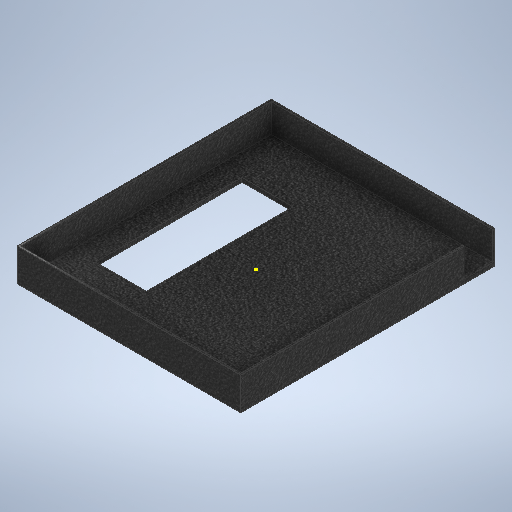
# Autodesk Inventor part: kotak_v2
Saved by Autodesk Inventor 2025.2 (Build 292293000, 293)
## iProperties
Created: 2025-02-11
Part Number: kotak_v2
Material: Generic
Document SubType Name: Modeling
Designer: ACER
Density: 1 g/cm^3
Appearance: Black Cast
Author: ACER
Autodesk Inventor part; units mm, degrees
ref_plane "YZ Plane" through (0, 0, 0) normal (1, 0, 0) x (0, 1, 0)
ref_plane "XZ Plane" through (0, 0, 0) normal (0, 1, 0) x (-1, 0, 0)
ref_plane "XY Plane" through (0, 0, 0) normal (0, 0, 1) x (1, 0, 0)
sketch "Sketch1" plane through (0, 0, 0) normal (0, 1, 0) x (-1, 0, 0)
  line L0 (-55, 62.5) -> (55, 62.5)
  line L1 (55, 62.5) -> (55, -62.5)
  line L2 (55, -62.5) -> (-55, -62.5)
  line L3 (-55, -62.5) -> (-55, 62.5)
  line L4 (-55, 62.5) -> (55, -62.5) construction
  line L5 (55, 62.5) -> (-55, -62.5) construction
  point P0 (0, 0)
  dimension "d0" = 125
  dimension "d1" = 110
  constraints: 12 end point, 2 midpoint, 2 parallel, 1 horizontal, 1 perpendicular
  measures "d0" distance of L0.end L1.end
  measures "d1" distance of L0.start L0.end
extrude "Extrusion1" add sketch "Sketch1" along normal blind 16
sketch "Sketch2" plane through (0, 16, 0) normal (0, 1, 0) x (1, 0, 0)
  line L0 (54, -61.5) -> (-54, -61.5)
  line L1 (-54, -61.5) -> (-54, 61.5)
  line L2 (-54, 61.5) -> (54, 61.5)
  line L3 (54, 61.5) -> (54, -61.5)
  line L4 (54, -61.5) -> (-54, 61.5) construction
  line L5 (-54, -61.5) -> (54, 61.5) construction
  point P0 (0, 0)
  dimension "d4" = 123
  dimension "d5" = 108
  constraints: 12 end point, 2 midpoint, 2 parallel, 1 horizontal, 1 perpendicular
  measures "d4" distance of L0.end L1.end
  measures "d5" distance of L0.start L0.end
extrude "Extrusion2" cut sketch "Sketch2" against normal blind 14
sketch "Sketch3" plane through (0, 2, 0) normal (0, 1, 0) x (1, 0, 0)
  point P0 (0, 0)
sketch "Sketch4" plane through (0, 2, 0) normal (0, 1, 0) x (1, 0, 0)
  line L0 (-17.8843, -36) -> (-42.8843, -36)
  line L1 (-42.8843, -36) -> (-42.8843, 36)
  line L2 (-42.8843, 36) -> (-17.8843, 36)
  line L3 (-17.8843, 36) -> (-17.8843, -36)
  line L4 (-17.8843, -36) -> (-42.8843, 36) construction
  line L5 (-42.8843, -36) -> (-17.8843, 36) construction
  point P0 (0, 0)
  point P1 (-30.3843, 0)
  dimension "d8" = 72
  dimension "d9" = 25
  constraints: 12 end point, 2 midpoint, 2 parallel, 1 horizontal, 1 perpendicular
  measures "d8" distance of L0.end L1.end
  measures "d9" distance of L0.start L0.end
extrude "Extrusion3" cut sketch "Sketch4" against normal blind 14
sketch "Sketch5" plane through (54, 16, -61.5) normal (-1, 0, 0) x (0, 0, 1)
  point P0 (61.5, -16)
sketch "Sketch6" plane through (54, 16, -61.5) normal (-1, 0, 0) x (0, 0, 1)
  line L0 (0, 0) -> (0, -14) projected
  line L1 (0, -14) -> (123, -14) projected
  line L2 (0, 0) -> (14, 0)
  line L3 (14, 0) -> (14, -14)
  line L4 (14, -14) -> (0, -14)
  line L5 (0, -14) -> (0, 0)
  point P0 (61.5, -16)
  dimension "d12" = 14
  dimension "d13" = 123
  dimension "d14" = 14
  constraints: 8 end point, 2 parallel, 1 horizontal, 1 perpendicular, 1 point on line
  measures "d12" distance of L2.end L3.end
  measures "d13" distance of L0.end L1.end
  measures "d14" distance of L0.start L2.end
extrude "Extrusion4" cut sketch "Sketch6" against normal blind 14
body "Solid1"
